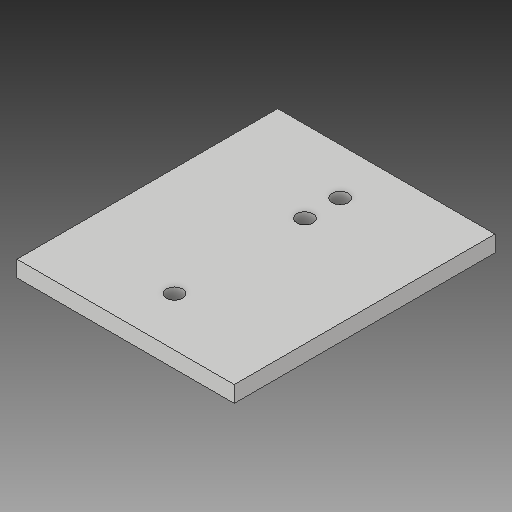
# Autodesk Inventor part: support-lanceur
Saved by Autodesk Inventor 2019 (Build 230136000, 136)
## iProperties
Created: 2018-04-06
Part Number: support-lanceur
Material: Générique
Document SubType Name: Modeling
Designer: franc
Density: 1 g/cm^3
Appearance: Par défaut
Author: franc
Autodesk Inventor part; units mm, degrees
ref_plane "YZ Plane" through (0, 0, 0) normal (1, 0, 0) x (0, 1, 0)
ref_plane "XZ Plane" through (0, 0, 0) normal (0, 1, 0) x (-1, 0, 0)
ref_plane "XY Plane" through (0, 0, 0) normal (0, 0, 1) x (1, 0, 0)
sketch "Sketch1" plane through (0, 0, 0) normal (0, 1, 0) x (-1, 0, 0)
  line L0 (13.7931, -3.0345) -> (-26.2069, -3.0345)
  line L1 (-26.2069, -3.0345) -> (-26.2069, -51.0345)
  line L2 (-26.2069, -51.0345) -> (13.7931, -51.0345)
  line L3 (13.7931, -51.0345) -> (13.7931, -3.0345)
  circle A0 centre (-6.2069, -12.0345) radius 1.5
  circle A1 centre (-6.2069, -42.5345) radius 1.5
  circle A2 centre (-6.2069, -36.0345) radius 1.5
  point P0 (0, 0)
  dimension "d0" = 48
  dimension "d1" = 40
  dimension "d2" = 3
  dimension "d4" = 20
  dimension "d7" = 8.5
  dimension "d8" = 15
  dimension "d9" = 3
  dimension "d10" = 3
  dimension "d11" = 20
  dimension "d12" = 20
  dimension "d13" = 9
  constraints: 8 end point, 3 centre point, 2 parallel, 1 horizontal, 1 perpendicular
  measures "d0" distance of L2.end L0.start
  measures "d1" distance of L0.start L0.end
  measures "d2" diameter of A0
  measures "d4" distance from line of L3 A0.centre
  measures "d7" distance from line of L2 A1.centre
  measures "d8" distance from line of L2 A2.centre
  measures "d9" diameter of A1
  measures "d10" diameter of A2
  measures "d11" distance from line of L1 A1.centre
  measures "d12" distance from line of L1 A2.centre
  measures "d13" distance from line of L0 A0.centre
extrude "Extrusion1" add sketch "Sketch1" along normal blind 3
equation "\"d5\" = d9"
body "Solid1"
